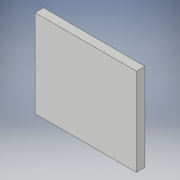
# Autodesk Inventor part: 空雞補底
Saved by Autodesk Inventor 2019 (Build 230136000, 136)
## iProperties
Created: 2019-01-19
Part Number: 空雞補底
Material: 一般
Document SubType Name: Modeling
Designer: j13tw
Density: 1 g/cm^3
Appearance: 預設
Author: j13tw
Autodesk Inventor part; units mm, degrees
ref_plane "YZ Plane" through (0, 0, 0) normal (1, 0, 0) x (0, 1, 0)
ref_plane "XZ Plane" through (0, 0, 0) normal (0, 1, 0) x (-1, 0, 0)
ref_plane "XY Plane" through (0, 0, 0) normal (0, 0, 1) x (1, 0, 0)
sketch "草圖1" plane through (0, 0, 0) normal (0, 0, 1) x (1, 0, 0)
  line L0 (0, 0) -> (59.65, 0)
  line L1 (59.65, 0) -> (59.65, 51.48)
  line L2 (59.65, 51.48) -> (0, 51.48)
  line L3 (0, 51.48) -> (0, 0)
  dimension "d0" = 59.65
  dimension "d1" = 51.48
  constraints: 8 end point, 2 parallel, 1 horizontal, 1 perpendicular
  measures "d0" distance of L1.end L2.end
  measures "d1" distance of L0.end L1.end
extrude "擠出1" add sketch "草圖1" along normal blind 5
